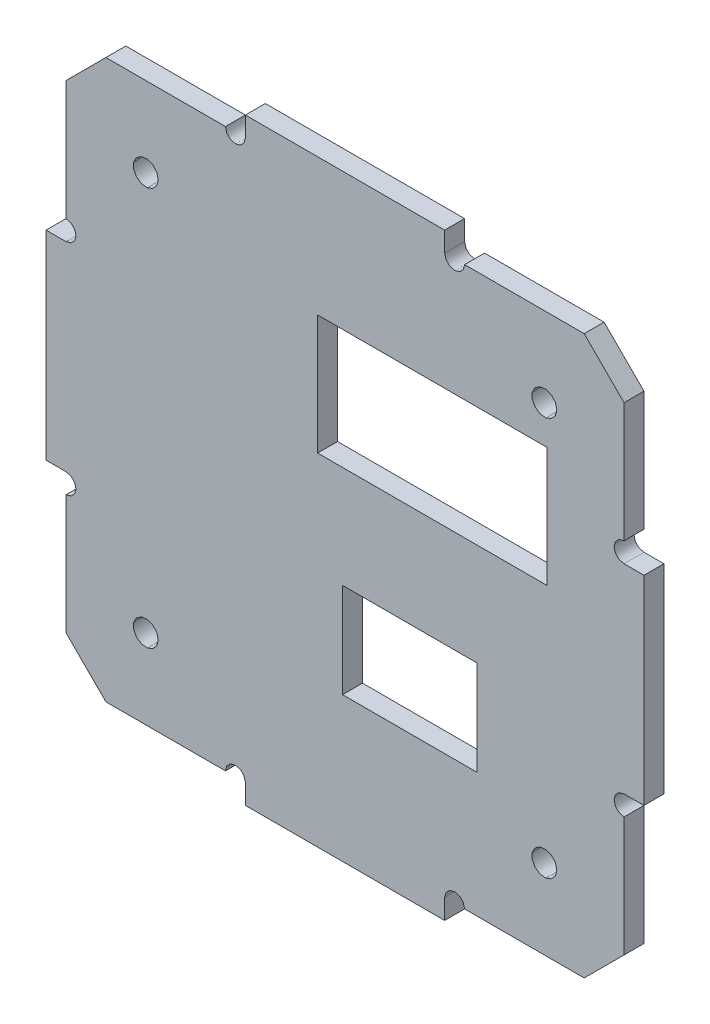
# Autodesk Inventor part: Tapa Enchufes
Saved by Autodesk Inventor 2017 (Build 210142000, 142)
## iProperties
Part Number: Tapa Enchufes
Material: Genérico
Document SubType Name: Modeling
Designer: Leo
Density: 1 g/cm^3
Appearance: Valor por defecto
Description: Aluminio compuesto routeado CNC
Author: Leo
Autodesk Inventor part; units mm, degrees
ref_plane "YZ Plane" through (0, 0, 0) normal (1, 0, 0) x (0, 1, 0)
ref_plane "XZ Plane" through (0, 0, 0) normal (0, 1, 0) x (-1, 0, 0)
ref_plane "XY Plane" through (0, 0, 0) normal (0, 0, 1) x (1, 0, 0)
sketch "Boceto1" plane through (0, 0, 0) normal (0, 0, 1) x (1, 0, 0)
  line L0 (-60, 20) -> (-60, -20)
  line L1 (-60, -20) -> (-56, -20)
  arc A0 (-56, -24) -> (-56, -20) centre (-56, -22) ccw
  line L2 (-56, -24) -> (-56, -48)
  line L3 (-56, -48) -> (-48, -56)
  line L4 (-48, -56) -> (-24, -56)
  arc A1 (-20, -56) -> (-24, -56) centre (-22, -56) ccw
  line L5 (-20, -56) -> (-20, -60)
  line L6 (-20, -60) -> (20, -60)
  line L7 (20, -60) -> (20, -56)
  arc A2 (24, -56) -> (20, -56) centre (22, -56) ccw
  line L8 (24, -56) -> (48, -56)
  line L9 (48, -56) -> (56, -48)
  line L10 (27.1297, 0) -> (-27.1297, 0) construction
  line L11 (0, -24.7936) -> (0, 24.7936) construction
  arc A3 (-56, 20) -> (-56, 24) centre (-56, 22) ccw
  line L12 (-56, 24) -> (-56, 48)
  line L13 (-56, 48) -> (-48, 56)
  line L14 (-48, 56) -> (-24, 56)
  arc A4 (-24, 56) -> (-20, 56) centre (-22, 56) ccw
  line L15 (-20, 56) -> (-20, 60)
  line L16 (-20, 60) -> (20, 60)
  line L17 (20, 60) -> (20, 56)
  arc A5 (20, 56) -> (24, 56) centre (22, 56) ccw
  line L18 (24, 56) -> (48, 56)
  line L19 (48, 56) -> (56, 48)
  line L20 (-56, 20) -> (-60, 20)
  line L21 (60, 20) -> (60, -20)
  line L22 (60, -20) -> (56, -20)
  arc A6 (56, -20) -> (56, -24) centre (56, -22) ccw
  line L23 (56, -24) -> (56, -48)
  line L24 (56, 24) -> (56, 48)
  arc A7 (56, 24) -> (56, 20) centre (56, 22) ccw
  line L25 (56, 20) -> (60, 20)
  circle A8 centre (40, -40) radius 2.5
  circle A9 centre (40, 40) radius 2.5
  circle A10 centre (-40, -40) radius 2.5
  circle A11 centre (-40, 40) radius 2.5
  line L26 (40.5, 8.5) -> (40.5, 32.5)
  line L27 (40.5, 32.5) -> (-5.5, 32.5)
  line L28 (-5.5, 32.5) -> (-5.5, 8.5)
  line L29 (-5.5, 8.5) -> (40.5, 8.5)
  line L30 (-18, 36) -> (-18, 5) construction
  line L31 (-18, 5) -> (53, 5) construction
  line L32 (53, 5) -> (53, 36) construction
  line L33 (53, 36) -> (-18, 36) construction
  line L34 (26.5, -12) -> (-0.5, -12)
  line L35 (-0.5, -12) -> (-0.5, -31)
  line L36 (-0.5, -31) -> (26.5, -31)
  line L37 (26.5, -31) -> (26.5, -12)
  point P0 (0, 0)
  point P1 (0, 0)
  point P2 (-60, 0)
  point P3 (0, 60)
  point P4 (17.5, 36)
  point P5 (17.5, 32.5)
  point P6 (53, 20.5)
  point P7 (40.5, 20.5)
  dimension "d0" = 40
  dimension "d1" = 4
  dimension "d2" = 2
  dimension "d3" = 112
  dimension "d4" = 120
  dimension "d5" = 4
  dimension "d6" = 8
  dimension "d7" = 5
  dimension "d8" = 80
  dimension "d9" = 80
  dimension "d10" = 24
  dimension "d11" = 46
  dimension "d12" = 31
  dimension "d13" = 71
  dimension "d14" = 3
  dimension "d15" = 20
  dimension "d16" = 19
  dimension "d17" = 27
  dimension "d18" = 5
  dimension "d19" = 24
  constraints: 76 end point, 28 symmetric about line, 16 point on circle, 13 point on line, 12 centre point, 11 perpendicular, 8 midpoint, 7 parallel, 5 horizontal, 3 tangent, 2 equal radius, 2 horizontal alignment, 2 vertical, 1 coincident, 1 vertical alignment, 8 other
  measures "d0" distance of L0.start L0.end
  measures "d1" distance between parallel lines of L2 L0
  measures "d2" radius of A3
  measures "d3" distance between parallel lines of L24 L12
  measures "d4" distance between parallel lines of L6 L16
  measures "d5" distance between parallel lines of L16 L18
  measures "d6" horizontal distance of L8.end L9.end
  measures "d7" diameter of A8
  measures "d8" distance of A9.centre A8.centre
  measures "d9" distance of A10.centre A8.centre
  measures "d10" distance of L26.start L26.end
  measures "d11" distance of L26.end L27.end
  measures "d12" distance of L30.start L30.end
  measures "d13" distance of L30.end L31.end
  measures "d14" distance between parallel lines of L24 L32
  measures "d15" distance between parallel lines of L18 L33
  measures "d16" distance of L34.end L35.end
  measures "d17" distance of L34.start L34.end
  measures "d18" distance between parallel lines of L35 L28
  measures "d19" diameter of L34 L10
extrude "Extrusión1" add sketch "Boceto1" along normal blind 4
equation "\"d5\" = d1"
equation "\"d9\" = d8"
